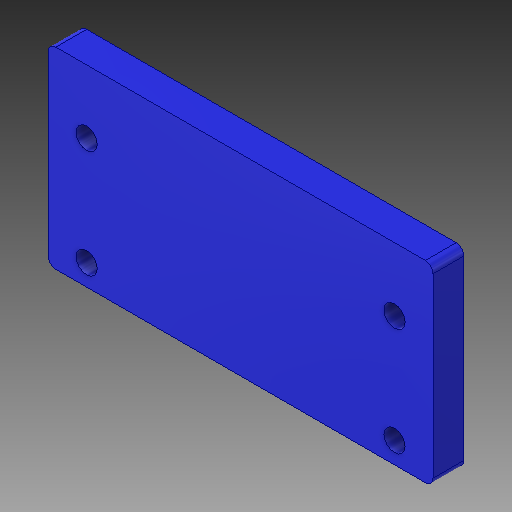
# Autodesk Inventor part: Piastra collegamento asse - pistone
Saved by Autodesk Inventor 2018 (Build 220112000, 112)
## iProperties
Created: 2020-06-01
Part Number: Piastra collegamento asse - pistone
Material: Generico
Document SubType Name: Modeling
Designer: Francesco
Density: 1 g/cm^3
Appearance: Blu - Pittura muro - Lucida
Author: Francesco
Autodesk Inventor part; units mm, degrees
ref_plane "YZ Plane" through (0, 0, 0) normal (1, 0, 0) x (0, 1, 0)
ref_plane "XZ Plane" through (0, 0, 0) normal (0, 1, 0) x (-1, 0, 0)
ref_plane "XY Plane" through (0, 0, 0) normal (0, 0, 1) x (1, 0, 0)
sketch "Schizzo1" plane through (0, 0, 0) normal (0, 0, 1) x (1, 0, 0)
  line L0 (-50, 25) -> (50, 25)
  line L1 (50, 25) -> (50, -25)
  line L2 (50, -25) -> (-50, -25)
  line L3 (-50, -25) -> (-50, 25)
  line L4 (-50, 25) -> (50, -25) construction
  line L5 (50, 25) -> (-50, -25) construction
  point P0 (0, 0)
  dimension "d0" = 100
  dimension "d1" = 50
  constraints: 12 end point, 2 midpoint, 2 parallel, 1 horizontal, 1 perpendicular
  measures "d0" distance of L1.end L2.end
  measures "d1" distance of L0.end L1.end
extrude "Estrusione1" add sketch "Schizzo1" along normal blind 8
fillet "Raccordo1" radius 2 4 edges at (-50, 25, 4) (50, 25, 4) (50, -25, 4) (-50, -25, 4)
sketch "Schizzo2" plane through (0, 0, 8) normal (0, 0, 1) x (1, 0, 0)
  circle A0 centre (-40, -19.5) radius 2.067
  line L0 (-48, -25) -> (48, -25) projected
  line L1 (-50, 23) -> (-50, -23) projected
  line L2 (50, -23) -> (50, 23) projected
  point P0 (0, 0)
  point P1 (-40, 8.5)
  point P2 (40, 8.5)
  point P3 (40, -19.5)
  dimension "d13" = 28
  dimension "d16" = 5.5
  dimension "d17" = 10
  dimension "d18" = 10
  constraints: 2 horizontal alignment, 2 vertical alignment, 1 centre point, 1 coincident
  measures "d13" distance of point (-40, 8.5) point (-40, -19.5)
  measures "d16" distance from line of L0 point (-40, -19.5)
  measures "d17" distance from line of L1 point (-40, -19.5)
  measures "d18" distance from line of L2 point (40, -19.5)
hole "Foro1" at (-40, -19.5, 8) at (-40, 8.5, 8) at (40, 8.5, 8) at (40, -19.5, 8) direction (0, 0, -1) diameter 5.5 end through all clearance for "Vite a testa esagonale con calotta ISO 24017" size "M5" standard "ISO"
